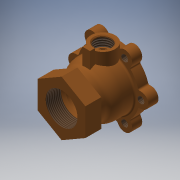
# Autodesk Inventor part: Body
Saved by Autodesk Inventor 2018 (Build 220112000, 112)
## iProperties
Shininess: 64.0
Length Units: 11269
Angle Units: 11279
Time Units: 11290
Mass Units: 11283
Length Display Precision: 3
Angle Display Precision: 2
Compacted: True
Part Number: Body
Document SubType Name: Modeling
Created: 2003-04-19
Designer: James M. Leake
Material: Bronze, Soft Tin
Density: 8.874 g/cm^3
Appearance: Bronze - Satin
Density: 0.0
Volumn: 0.0
Area: 0.0
PropertySet Name: Model Information
Control State: 0
Master: False
Checked Out: False
Author: James M. Leake
Autodesk Inventor part; units mm, degrees
note: some values were not read from the file. Chosen so that the rebuilt part matches the saved one: direction of "Hole4".
ref_plane "YZ Plane" through (0, 0, 0) normal (1, 0, 0) x (0, 1, 0)
sketch "Sketch1" plane through (0, 0, 0) normal (0, 0, 1) x (1, 0, 0)
  line L0 (-3.7, 0) -> (48.1, 0) projected
  line L1 (0, -6.8) -> (0, 88.4) projected
  line L2 (19, 0) -> (19, 18)
  line L3 (19, 18) -> (16, 21)
  line L4 (16, 21) -> (16, 24)
  line L5 (16, 24) -> (23, 24)
  line L6 (23, 24) -> (23, 33)
  arc A0 (23, 33) -> (28.5, 38.5) centre (23, 38.5) ccw
  line L7 (28.5, 38.5) -> (28.5, 68)
  line L8 (28.5, 68) -> (37, 68)
  line L9 (37, 68) -> (37, 56)
  line L10 (37, 56) -> (31.5, 56)
  line L11 (31.5, 56) -> (31.5, 42.3631)
  arc A1 (28.4062, 31.1135) -> (31.5, 42.3631) centre (9.5, 42.3631) ccw
  arc A2 (28.4062, 31.1135) -> (27, 26) centre (37, 26) ccw
  line L12 (27, 26) -> (27, 0)
  line L13 (27, 0) -> (19, 0)
  point P0 (0, 0)
  dimension "d0" = 54
  dimension "d1" = 38
  dimension "d2" = 32
  dimension "d3" = 46
  dimension "d4" = 57
  dimension "d5" = 63
  dimension "d6" = 74
  dimension "d7" = 12
  dimension "d8" = 68
  dimension "d9" = 26
  dimension "d10" = 18
  dimension "d11" = 21
  dimension "d12" = 24
  dimension "d13" = 33
  dimension "d14" = 22
  dimension "d15" = 10
  constraints: 24 end point, 8 perpendicular, 6 point on circle, 4 tangent, 3 centre point, 3 parallel, 3 point on line
  measures "d0" diameter of L12 L1
  measures "d1" diameter of L2 L1
  measures "d2" diameter of L4 L1
  measures "d3" diameter of L6 L1
  measures "d4" diameter of L7 L1
  measures "d5" diameter of L11 L1
  measures "d6" diameter of L9 L1
  measures "d7" distance of L8.end L9.end
  measures "d8" distance between parallel lines of L8 L13
  measures "d9" distance of L12.start L12.end
  measures "d10" distance of L2.start L2.end
  measures "d11" distance from line of L13 L3.end
  measures "d12" distance between parallel lines of L13 L5
  measures "d13" distance from line of L13 L6.end
  measures "d14" radius of A1
  measures "d15" radius of A2
revolve "Revolution1" add sketch "Sketch1" angle 360 about axis through (0, -10, 0) along (0, 1, 0)
sketch "Sketch2" plane through (0, 0, 0) normal (0, -1, 0) x (1, 0, 0)
  circle A0 centre (0, 0) radius 27 projected
  line L0 (-44.4, 0) -> (59.2, 0) projected
  line L1 (0, -44.4) -> (0, 59.2) projected
  line L2 (0, -32.909) -> (-28.5, -16.4545)
  line L3 (-28.5, -16.4545) -> (-28.5, 16.4545)
  line L4 (-28.5, 16.4545) -> (0, 32.909)
  line L5 (0, 32.909) -> (28.5, 16.4545)
  line L6 (28.5, 16.4545) -> (28.5, -16.4545)
  line L7 (28.5, -16.4545) -> (0, -32.909)
  dimension "d17" = 57
  constraints: 12 end point, 1 coincident, 1 point on line, 11 other
  measures "d17" distance between parallel lines of L6 L3
extrude "Extrusion1" add sketch "Sketch2" against normal blind 19 contours L0 L6 L7 L1 A0 | A0 L1 L5 L6 L0 | A0 L0 L3 L4 L1 | L1 L2 L3 L0 A0
sketch "Sketch3" plane through (0, 68, 0) normal (0, 1, 0) x (1, 0, 0)
  circle A0 centre (0, 0) radius 37 projected
  line L0 (-44.4, 0) -> (59.2, 0) projected
  line L1 (0, 44.4) -> (0, -59.2) projected
  line L2 (35.8887, 9) -> (39, 9)
  arc A1 (39, -9) -> (39, 9) centre (39, 0) ccw
  line L3 (39, -9) -> (35.8887, -9)
  dimension "d20" = 78
  dimension "d21" = 9
  constraints: 4 end point, 4 point on circle, 2 tangent, 1 centre point, 1 parallel, 1 perpendicular, 1 other
  measures "d20" diameter of A1.centre L1
  measures "d21" radius of A1
extrude "Extrusion2" add sketch "Sketch3" against normal blind 12 contours L0 A1 L3 A0 | A0 L2 A1 L0
fillet "Fillet1" radius 2 2 edges at (35.8887, 62, 9) (35.8887, 62, -9)
sketch "Sketch4" plane through (39, 68, 0) normal (0, 1, 0) x (1, 0, 0)
  arc A0 (0, -9) -> (0, 9) centre (0, 0) ccw projected
  constraints: 1 coincident
hole "Hole1" at (39, 68, 0) direction (0, -1, 0) diameter 8 end through all thread size "M8x1.25" class "6H" standard "ANSI Metric M Profile"
pattern_circular "Circular Pattern1" count 6 over 360 about axis through (0, 9, 0) along (0, -1, 0) of "Extrusion2", "Hole1", "Fillet1"
thread "Thread1" size "M39x2" class "6H" standard "ANSI Metric M Profile" full length
fillet "Fillet2" radius 2 1 edges at (-31.5, 56, 0)
ref_plane "Work Plane1" through (0, 0, 44) normal (0, 0, 1) x (1, 0, 0)
sketch "Sketch5" plane through (0, 0, 44) normal (0, 0, 1) x (1, 0, 0)
  line L0 (0, -6.8) -> (0, 88.4) projected
  line L1 (-8.7111, 68) -> (8.7111, 68) projected
  circle A0 centre (0, 49.5) radius 14.5
  dimension "d39" = 29
  dimension "d40" = 18.5
  constraints: 1 centre point, 1 point on line
  measures "d39" diameter of A0
  measures "d40" distance from line of L1 A0.centre
extrude "Extrusion3" add sketch "Sketch5" against normal up to next
sketch "Sketch6" plane through (0, 49.5, 44) normal (0, 0, 1) x (1, 0, 0)
  circle A0 centre (0, 0) radius 14.5 projected
  constraints: 1 coincident
hole "Hole4" at (0, 49.5, 44) direction (0, 0, -1) diameter 16 end up to surface counterbore diameter 20 counterbore depth 12
chamfer "Chamfer2" distance 1 angle 45 1 edges at (0, 59.5, 44) measured on face at (12.8352, 47.9415, 44)
thread "Thread3" size "M20x2.5" class "6H" standard "ANSI Metric M Profile" length 10
ref_plane "Work Plane3" through (0, 0, 47) normal (0, 0, 1) x (1, 0, 0)
sketch "Sketch8" plane through (0, 0, 47) normal (0, 0, 1) x (1, 0, 0)
  line L0 (0, -6.8) -> (0, 88.4) projected
  line L1 (-4.5, 35.5) -> (4.5, 35.5)
  line L2 (4.5, 35.5) -> (4.5, 29.5)
  line L3 (4.5, 29.5) -> (-4.5, 29.5)
  line L4 (-4.5, 29.5) -> (-4.5, 35.5)
  line L5 (-8.7111, 68) -> (8.7111, 68) projected
  dimension "d80" = 32.5
  dimension "d81" = 6
  dimension "d82" = 4.5
  dimension "d83" = 9
  constraints: 8 end point, 2 parallel, 1 horizontal, 1 perpendicular
  measures "d80" distance between parallel lines of L5 L1
  measures "d81" distance of L3.end L1.start
  measures "d82" distance between parallel lines of L0 L4
  measures "d83" distance of L2.end L3.end
extrude "Extrusion5" add sketch "Sketch8" against normal up to next
body "Solid1"
